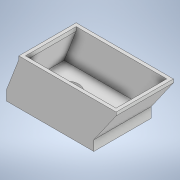
# Autodesk Inventor part: Übersetzungsbox_2
Saved by Autodesk Inventor 2021 (Build 250183000, 183)
## iProperties
Created: 2021-01-10
Part Number: Übersetzungsbox_2
Material: Generisch
Document SubType Name: Modeling
Designer: Ctroi
Density: 1 g/cm^3
Appearance: Vorgabe
Author: Ctroi
Autodesk Inventor part; units mm, degrees
ref_plane "YZ Plane" through (0, 0, 0) normal (1, 0, 0) x (0, 1, 0)
ref_plane "XZ Plane" through (0, 0, 0) normal (0, 1, 0) x (-1, 0, 0)
ref_plane "XY Plane" through (0, 0, 0) normal (0, 0, 1) x (1, 0, 0)
sketch "Skizze1" plane through (0, 0, 0) normal (0, 1, 0) x (-1, 0, 0)
  line L0 (-26, -17.1) -> (26, -17.1)
  line L1 (26, -17.1) -> (26, 17.1)
  line L2 (26, 17.1) -> (-26, 17.1)
  line L3 (-26, 17.1) -> (-26, -17.1)
  line L4 (0, -23.94) -> (0, 23.94) projected
  line L5 (-36.4, 0) -> (36.4, 0) projected
  point P0 (0, 0)
  dimension "d0" = 52
  dimension "d1" = 34.2
  constraints: 8 end point, 2 parallel, 1 horizontal, 1 perpendicular, 2 other
  measures "d0" distance of L1.end L2.end
  measures "d1" distance of L0.end L1.end
extrude "Extrusion1" add sketch "Skizze1" along normal blind 6
ref_plane "Arbeitsebene1" through (0, 25, 0) normal (0, 1, 0) x (1, 0, 0)
sketch "Skizze2" plane through (0, 25, 0) normal (0, 1, 0) x (1, 0, 0)
  line L0 (26, 17.1) -> (-26, 17.1) projected
  line L1 (-18.7, 17.1) -> (39.3, 17.1)
  line L2 (39.3, 17.1) -> (39.3, -17.1)
  line L3 (39.3, -17.1) -> (-18.7, -17.1)
  line L4 (-18.7, -17.1) -> (-18.7, 17.1)
  line L5 (-26, 17.1) -> (-26, -17.1) projected
  point P0 (0, 0)
  dimension "d5" = 58
  dimension "d6" = 34.2
  dimension "d7" = 7.3
  constraints: 8 end point, 2 parallel, 1 horizontal, 1 perpendicular, 1 point on line
  measures "d5" distance of L2.end L3.end
  measures "d6" distance of L1.end L2.end
  measures "d7" distance between parallel lines of L5 L4
extrude "Extrusion2" add sketch "Skizze2" along normal blind 2
loft "Erhebung1" add section 1 edges at (-26, 6, 0) (0, 6, 17.1) (26, 6, 0) (0, 6, -17.1) section 2 edges at (39.3, 25, 0) (10.3, 25, 17.1) (-18.7, 25, 0) (10.3, 25, -17.1)
shell "Wandung1" thickness 2 removed faces 1 at (0.6333, 27, -5.7)
sketch "Skizze7" plane through (-24, 2, 15.1) normal (0, 1, 0) x (1, 0, 0)
  line L0 (-2, 32.2) -> (-2, -2) projected
  line L1 (50, 32.2) -> (-2, 32.2) projected
  line L2 (-2, -2) -> (50, -2)
  line L3 (50, -2) -> (50, 32.2)
  line L4 (50, 32.2) -> (-2, 32.2)
  line L5 (-2, 32.2) -> (-2, -2)
  line L6 (48, 0) -> (0, 0)
  line L7 (0, 0) -> (0, 30.2)
  line L8 (0, 30.2) -> (48, 30.2)
  line L9 (48, 30.2) -> (48, 0)
  point P0 (24, 15.1)
  dimension "d28" = 2
  constraints: 16 end point, 4 parallel, 2 perpendicular, 1 horizontal, 3 other
  measures "d28" distance between parallel lines of L2 L6
extrude "Extrusion5" add sketch "Skizze7" along normal blind 4 contours L6 L7 L8 L9
sketch "Skizze8" plane through (-24, 6, 15.1) normal (0, 1, 0) x (1, 0, 0)
  circle A0 centre (16.7, 15.1) radius 7.25
  line L0 (-2, 32.2) -> (-2, -2) projected
  line L1 (50, 32.2) -> (-2, 32.2) projected
  point P0 (24, 15.1)
  dimension "d31" = 14.5
  dimension "d32" = 18.7
  dimension "d33" = 17.1
  constraints: 1 centre point
  measures "d31" diameter of A0
  measures "d32" distance from line of L0 A0.centre
  measures "d33" distance from line of L1 A0.centre
extrude "Extrusion7" cut sketch "Skizze8" against normal blind 4
sketch "Skizze9" plane through (-7.3, 2, 0) normal (0, 1, 0) x (1, 0, 0)
  circle A0 centre (0, 0) radius 5.25
  point P0 (7.3, 0)
  dimension "d38" = 10.5
  constraints: 1 centre point
  measures "d38" diameter of A0
extrude "Extrusion8" cut sketch "Skizze9" against normal up to surface (2 mm away)
